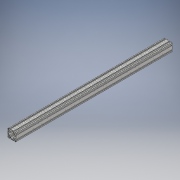
# Autodesk Inventor part: 60x60x1100 Profil
Saved by Autodesk Inventor 2019 (Build 230136000, 136)
## iProperties
Created: 2021-05-01
Part Number: 60x60x1100 Profil
Material: Generic
Document SubType Name: Modeling
Designer: Michael Sumper
Density: 1 g/cm^3
Appearance: Default
Author: Michael Sumper
Autodesk Inventor part; units mm, degrees
ref_plane "YZ Plane" through (0, 0, 0) normal (1, 0, 0) x (0, 1, 0)
ref_plane "XZ Plane" through (0, 0, 0) normal (0, 1, 0) x (-1, 0, 0)
ref_plane "XY Plane" through (0, 0, 0) normal (0, 0, 1) x (1, 0, 0)
sketch "Skizze1" plane through (0, 0, 0) normal (0, 0, 1) x (1, 0, 0)
  line L0 (-30, -30) -> (30, 30) construction
  line L1 (30, -30) -> (-30, 30) construction
  line L2 (-15, -15) -> (15, -15) construction
  line L3 (15, -15) -> (15, 15) construction
  line L4 (15, 15) -> (-15, 15) construction
  line L5 (-15, 15) -> (-15, -15) construction
  line L6 (-15, -15) -> (15, 15) construction
  line L7 (15, -15) -> (-15, 15) construction
  circle A0 centre (-15, 15) radius 2.5
  circle A1 centre (15, 15) radius 2.5
  circle A2 centre (15, -15) radius 2.5
  circle A3 centre (-15, -15) radius 2.5
  line L8 (-18.5, 20.25) -> (-11.5, 20.25)
  line L9 (-9.75, 17.702) -> (-9.75, 9.75)
  line L10 (-9.75, 9.75) -> (-17.702, 9.75)
  line L11 (-20.25, 11.5) -> (-20.25, 18.5)
  line L12 (-20.25, 20.25) -> (-9.75, 9.75) construction
  line L13 (-9.75, 20.25) -> (-20.25, 9.75) construction
  line L14 (11.5, 20.25) -> (18.5, 20.25)
  line L15 (20.25, 18.5) -> (20.25, 11.5)
  line L16 (17.702, 9.75) -> (9.75, 9.75)
  line L17 (9.75, 9.75) -> (9.75, 17.702)
  line L18 (9.75, 20.25) -> (20.25, 9.75) construction
  line L19 (20.25, 20.25) -> (9.75, 9.75) construction
  line L20 (11.5, -20.25) -> (18.5, -20.25)
  line L21 (20.25, -18.5) -> (20.25, -11.5)
  line L22 (17.702, -9.75) -> (9.75, -9.75)
  line L23 (9.75, -9.75) -> (9.75, -17.702)
  line L24 (9.75, -20.25) -> (20.25, -9.75) construction
  line L25 (20.25, -20.25) -> (9.75, -9.75) construction
  line L26 (-18.5, -20.25) -> (-11.5, -20.25)
  line L27 (-9.75, -17.702) -> (-9.75, -9.75)
  line L28 (-9.75, -9.75) -> (-17.702, -9.75)
  line L29 (-20.25, -11.5) -> (-20.25, -18.5)
  line L30 (-20.25, -20.25) -> (-9.75, -9.75) construction
  line L31 (-9.75, -20.25) -> (-20.25, -9.75) construction
  arc A4 (-25, 30) -> (-30, 25) centre (-25, 25) ccw
  arc A5 (30, 25) -> (25, 30) centre (25, 25) ccw
  arc A6 (25, -30) -> (30, -25) centre (25, -25) ccw
  arc A7 (-30, -25) -> (-25, -30) centre (-25, -25) ccw
  line L32 (0, 30) -> (-11.5, 30) construction
  line L33 (-11.5, 30) -> (-11.5, 27)
  line L34 (-11.5, 27) -> (-8.5, 27)
  line L35 (-8.5, 27) -> (-8.5, 28.5)
  line L36 (-8.5, 28.5) -> (-3.25, 28.5)
  line L37 (-3.25, 28.5) -> (-11.5, 20.25)
  line L38 (-11.5, 30) -> (-15, 30) construction
  line L39 (-18.5, 30) -> (-18.5, 27)
  line L40 (-18.5, 27) -> (-21.5, 27)
  line L41 (-21.5, 27) -> (-21.5, 28.5)
  line L42 (-21.5, 28.5) -> (-26.75, 28.5)
  line L43 (-26.75, 28.5) -> (-18.5, 20.25)
  line L44 (-26.75, 28.5) -> (-15.0827, 28.5) construction
  line L45 (-28.5, -26.75) -> (-20.25, -18.5)
  line L46 (-28.5, -21.5) -> (-28.5, -26.75)
  line L47 (-27, -21.5) -> (-28.5, -21.5)
  line L48 (-27, -18.5) -> (-27, -21.5)
  line L49 (-30, -18.5) -> (-27, -18.5)
  line L50 (-30, -11.5) -> (-27, -11.5)
  line L51 (-27, -11.5) -> (-27, -8.5)
  line L52 (-27, -8.5) -> (-28.5, -8.5)
  line L53 (-28.5, -8.5) -> (-28.5, -3.25)
  line L54 (-28.5, -3.25) -> (-20.25, -11.5)
  line L55 (26.75, -28.5) -> (18.5, -20.25)
  line L56 (21.5, -28.5) -> (26.75, -28.5)
  line L57 (21.5, -27) -> (21.5, -28.5)
  line L58 (18.5, -27) -> (21.5, -27)
  line L59 (18.5, -30) -> (18.5, -27)
  line L60 (11.5, -30) -> (11.5, -27)
  line L61 (11.5, -27) -> (8.5, -27)
  line L62 (8.5, -27) -> (8.5, -28.5)
  line L63 (8.5, -28.5) -> (3.25, -28.5)
  line L64 (3.25, -28.5) -> (11.5, -20.25)
  line L65 (28.5, 26.75) -> (20.25, 18.5)
  line L66 (28.5, 21.5) -> (28.5, 26.75)
  line L67 (27, 21.5) -> (28.5, 21.5)
  line L68 (27, 18.5) -> (27, 21.5)
  line L69 (30, 18.5) -> (27, 18.5)
  line L70 (30, 11.5) -> (27, 11.5)
  line L71 (27, 11.5) -> (27, 8.5)
  line L72 (27, 8.5) -> (28.5, 8.5)
  line L73 (28.5, 8.5) -> (28.5, 3.25)
  line L74 (28.5, 3.25) -> (20.25, 11.5)
  line L75 (0, 30) -> (0, -30) construction
  line L76 (-28.5, 26.75) -> (-20.25, 18.5)
  line L77 (-28.5, 21.5) -> (-28.5, 26.75)
  line L78 (-27, 21.5) -> (-28.5, 21.5)
  line L79 (-27, 18.5) -> (-27, 21.5)
  line L80 (-30, 18.5) -> (-27, 18.5)
  line L81 (-30, 11.5) -> (-27, 11.5)
  line L82 (-27, 11.5) -> (-27, 8.5)
  line L83 (-27, 8.5) -> (-28.5, 8.5)
  line L84 (-28.5, 8.5) -> (-28.5, 3.25)
  line L85 (-28.5, 3.25) -> (-20.25, 11.5)
  line L86 (-26.75, -28.5) -> (-18.5, -20.25)
  line L87 (-21.5, -28.5) -> (-26.75, -28.5)
  line L88 (-21.5, -27) -> (-21.5, -28.5)
  line L89 (-18.5, -27) -> (-21.5, -27)
  line L90 (-18.5, -30) -> (-18.5, -27)
  line L91 (-11.5, -30) -> (-11.5, -27)
  line L92 (-11.5, -27) -> (-8.5, -27)
  line L93 (-8.5, -27) -> (-8.5, -28.5)
  line L94 (-8.5, -28.5) -> (-3.25, -28.5)
  line L95 (-3.25, -28.5) -> (-11.5, -20.25)
  line L96 (28.5, -26.75) -> (20.25, -18.5)
  line L97 (28.5, -21.5) -> (28.5, -26.75)
  line L98 (27, -21.5) -> (28.5, -21.5)
  line L99 (27, -18.5) -> (27, -21.5)
  line L100 (30, -18.5) -> (27, -18.5)
  line L101 (30, -11.5) -> (27, -11.5)
  line L102 (27, -11.5) -> (27, -8.5)
  line L103 (27, -8.5) -> (28.5, -8.5)
  line L104 (28.5, -8.5) -> (28.5, -3.25)
  line L105 (28.5, -3.25) -> (20.25, -11.5)
  line L106 (26.75, 28.5) -> (18.5, 20.25)
  line L107 (21.5, 28.5) -> (26.75, 28.5)
  line L108 (21.5, 27) -> (21.5, 28.5)
  line L109 (18.5, 27) -> (21.5, 27)
  line L110 (18.5, 30) -> (18.5, 27)
  line L111 (11.5, 30) -> (11.5, 27)
  line L112 (11.5, 27) -> (8.5, 27)
  line L113 (8.5, 27) -> (8.5, 28.5)
  line L114 (8.5, 28.5) -> (3.25, 28.5)
  line L115 (3.25, 28.5) -> (11.5, 20.25)
  line L116 (25, 30) -> (18.5, 30)
  line L117 (30, 18.5) -> (30, 25)
  line L118 (30, -25) -> (30, -18.5)
  line L119 (30, -11.5) -> (30, 11.5)
  line L120 (18.5, -30) -> (25, -30)
  line L121 (-25, -30) -> (-18.5, -30)
  line L122 (-11.5, -30) -> (11.5, -30)
  line L123 (-30, -18.5) -> (-30, -25)
  line L124 (-30, 25) -> (-30, 18.5)
  line L125 (-30, 11.5) -> (-30, -11.5)
  line L126 (11.5, 30) -> (-11.5, 30)
  line L127 (-18.5, 30) -> (-25, 30)
  line L128 (0, 30) -> (0, 26.3) construction
  line L129 (0, 26.3) -> (-1.152, 26.3)
  line L130 (0, 26.3) -> (1.152, 26.3)
  line L131 (1.152, 26.3) -> (9.75, 17.702)
  line L132 (-1.152, 26.3) -> (-9.351, 18.101)
  line L133 (-1.152, 26.3) -> (10.4431, 26.3) construction
  line L134 (-9.351, 18.101) -> (-9.75, 17.702)
  line L135 (-30, 0) -> (30, 0) construction
  line L136 (-26.3, -1.152) -> (-18.101, -9.351)
  line L137 (-18.101, -9.351) -> (-17.702, -9.75)
  line L138 (-26.3, 0) -> (-26.3, -1.152)
  line L139 (-26.3, 1.152) -> (-17.702, 9.75)
  line L140 (-26.3, -1.152) -> (-26.3, 10.4431) construction
  line L141 (-26.3, 0) -> (-26.3, 1.152)
  line L142 (1.152, -26.3) -> (9.351, -18.101)
  line L143 (9.351, -18.101) -> (9.75, -17.702)
  line L144 (0, -26.3) -> (1.152, -26.3)
  line L145 (-1.152, -26.3) -> (-9.75, -17.702)
  line L146 (1.152, -26.3) -> (-10.4431, -26.3) construction
  line L147 (0, -26.3) -> (-1.152, -26.3)
  line L148 (26.3, 1.152) -> (18.101, 9.351)
  line L149 (18.101, 9.351) -> (17.702, 9.75)
  line L150 (26.3, 0) -> (26.3, 1.152)
  line L151 (26.3, -1.152) -> (17.702, -9.75)
  line L152 (26.3, 1.152) -> (26.3, -10.4431) construction
  line L153 (26.3, 0) -> (26.3, -1.152)
  point P0 (0, 0)
  dimension "d0" = 60
  dimension "d1" = 60
  dimension "d2" = 30
  dimension "d3" = 30
  dimension "d4" = 5
  dimension "d5" = 5
  dimension "d6" = 5
  dimension "d7" = 5
  dimension "d8" = 10.5
  dimension "d9" = 10.5
  dimension "d10" = 10.5
  dimension "d11" = 10.5
  dimension "d12" = 10.5
  dimension "d13" = 10.5
  dimension "d14" = 10.5
  dimension "d15" = 10.5
  dimension "d16" = 5
  dimension "d17" = 5
  dimension "d18" = 11.5
  dimension "d19" = 3
  dimension "d20" = 3
  dimension "d21" = 1.5
  dimension "d22" = 5.25
  dimension "d23" = 45
  dimension "d24" = 7
  dimension "d25" = 3
  dimension "d26" = 3
  dimension "d27" = 1.5
  dimension "d28" = 5.25
  dimension "d29" = 45
  dimension "d32" = 360
  dimension "d36" = 360
  dimension "d38" = 3.7
  dimension "d39" = 1.152
  dimension "d40" = 1.152
  dimension "d41" = 135
  dimension "d42" = 135
  dimension "d45" = 360
  constraints: 308 end point, 28 parallel, 24 tangent, 19 horizontal, 19 perpendicular, 16 midpoint, 12 symmetric about line, 8 centre point, 8 point on circle, 6 point on line, 4 coincident, 2 equal length, 2 equal radius, 2 vertical, 233 other
  measures "d0" distance of L1.end L0.end
  measures "d1" distance of L0.end L1.start
  measures "d2" distance of L4.end L3.end
  measures "d3" distance of L3.end L2.end
  measures "d4" diameter of A0
  measures "d5" diameter of A1
  measures "d6" diameter of A2
  measures "d7" diameter of A3
  measures "d8" distance of L9.end L13.end
  measures "d9" distance of L13.start L9.end
  measures "d10" distance of L18.end L16.end
  measures "d11" distance of L19.start L18.end
  measures "d12" distance of L22.end L24.end
  measures "d13" distance of L24.end L25.start
  measures "d14" distance of L31.end L27.end
  measures "d15" distance of L27.end L31.start
  measures "d16" radius of A4
  measures "d17" radius of A5
  measures "d18" distance of L32.start L32.end
  measures "d19" distance of L32.end L33.end
  measures "d20" distance of L33.end L34.end
  measures "d21" distance of L34.end L35.end
  measures "d22" distance of L35.end L36.end
  measures "d23" angle of L36 L37
  measures "d24" distance of L32.end L39.start
  measures "d25" distance of L39.start L39.end
  measures "d26" distance of L39.end L40.end
  measures "d27" distance of L40.end L41.end
  measures "d28" distance of L41.end L42.end
  measures "d29" angle of L43 L44
  measures "d38" distance of L32.start L128.end
  measures "d39" distance of L128.end L129.end
  measures "d40" distance of L128.end L130.end
  measures "d41" angle of L130 L131
  measures "d42" angle of L132 L133
extrude "Extrusion1" add sketch "Skizze1" along normal blind 1100
